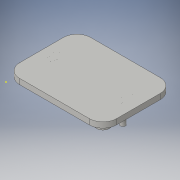
# Autodesk Inventor part: Router Bottom
Saved by Autodesk Inventor 2016 (Build 200138000, 138)
## iProperties
Created: 2016-01-12
Part Number: Router Bottom
Material: Generic
Document SubType Name: Modeling
Designer: Spooner
Density: 1 g/cm^3
Appearance: Default
Author: Spooner
Autodesk Inventor part; units mm, degrees
ref_plane "YZ Plane" through (0, 0, 0) normal (1, 0, 0) x (0, 1, 0)
ref_plane "XZ Plane" through (0, 0, 0) normal (0, 1, 0) x (-1, 0, 0)
ref_plane "XY Plane" through (0, 0, 0) normal (0, 0, 1) x (1, 0, 0)
sketch "Sketch1" plane through (0, 0, 0) normal (0, 1, 0) x (-1, 0, 0)
  line L0 (0, 0) -> (-90.17, 0)
  line L1 (-90.17, 0) -> (-90.17, -66.04)
  line L2 (-90.17, -66.04) -> (0, -66.04)
  line L3 (0, -66.04) -> (0, 0)
  dimension "d0" = 90.17
  dimension "d1" = 66.04
  constraints: 8 end point, 2 parallel, 1 horizontal, 1 perpendicular
  measures "d0" distance of L1.end L2.end
  measures "d1" distance of L0.end L1.end
extrude "Extrusion1" add sketch "Sketch1" along normal blind 5.08
sketch "Sketch2" plane through (0, 0, 0) normal (0, -1, 0) x (1, 0, 0)
  circle A0 centre (8.9218, -8.9217) radius 5.8738
  circle A1 centre (81.2483, -8.9218) radius 5.8738
  circle A2 centre (8.9217, -57.1183) radius 5.8738
  circle A3 centre (81.2483, -57.1183) radius 5.8738
  line L0 (0, 0) -> (90.17, 0) projected
  line L1 (0, -66.04) -> (0, 0) projected
  line L2 (90.17, -66.04) -> (0, -66.04) projected
  line L3 (90.17, 0) -> (90.17, -66.04) projected
  dimension "d4" = 11.7475
  dimension "d5" = 3.048
  dimension "d6" = 3.048
  dimension "d7" = 3.048
  dimension "d8" = 3.048
  constraints: 4 centre point, 3 equal radius, 2 horizontal alignment, 2 vertical alignment
  measures "d4" diameter of A0
  measures "d5" distance edge to line of A1 L0
  measures "d6" distance edge to line of A1 L3
  measures "d7" distance edge to line of A0 L1
  measures "d8" distance edge to line of A3 L2
extrude "Extrusion2" add sketch "Sketch2" along normal blind 2.5908 contours A0 | A1 | A2 | A3
sketch "Sketch3" plane through (0, 0, 0) normal (0, -1, 0) x (1, 0, 0)
  line L0 (78.6638, -30.099) -> (78.6638, -35.941) construction
  line L1 (73.5838, -30.099) -> (73.5838, -35.941)
  line L2 (83.7438, -35.941) -> (83.7438, -30.099)
  arc A0 (83.7438, -30.099) -> (73.5838, -30.099) centre (78.6638, -30.099) ccw
  arc A1 (73.5838, -35.941) -> (83.7438, -35.941) centre (78.6638, -35.941) ccw
  line L3 (11.5062, -30.099) -> (11.5062, -35.941) construction
  line L4 (6.4262, -30.099) -> (6.4262, -35.941)
  line L5 (16.5862, -35.941) -> (16.5862, -30.099)
  arc A2 (16.5862, -30.099) -> (6.4262, -30.099) centre (11.5062, -30.099) ccw
  arc A3 (6.4262, -35.941) -> (16.5862, -35.941) centre (11.5062, -35.941) ccw
  line L6 (90.17, 0) -> (90.17, -66.04) projected
  line L7 (0, -66.04) -> (0, 0) projected
  point P0 (78.6638, -33.02)
  point P1 (11.5062, -33.02)
  point P2 (90.17, -33.02)
  dimension "d11" = 6.4262
  dimension "d12" = 10.16
  dimension "d14" = 6.4262
  dimension "d15" = 16.002
  constraints: 16 end point, 8 point on circle, 8 tangent, 4 centre point, 3 midpoint, 3 parallel, 2 horizontal alignment, 2 vertical, 1 equal radius
  measures "d11" distance from line of L2 point (90.17, -33.02)
  measures "d12" distance from line of L1.end L2
  measures "d14" distance between parallel lines of L4 L7
extrude "Extrusion3" add sketch "Sketch3" along normal blind 4.064
sketch "Sketch4" plane through (0, -4.064, 0) normal (0, -1, 0) x (1, 0, 0)
  point P0 (0, 0)
sketch "Sketch5" plane through (0, -4.064, 0) normal (0, -1, 0) x (1, 0, 0)
  circle A0 centre (78.6638, -35.941) radius 4.1275
  circle A1 centre (11.5062, -35.941) radius 4.1275
  arc A2 (6.4262, -35.941) -> (16.5862, -35.941) centre (11.5062, -35.941) ccw projected
  arc A3 (73.5838, -35.941) -> (83.7438, -35.941) centre (78.6638, -35.941) ccw projected
  line L0 (11.5062, -35.941) -> (11.5062, -30.099) construction
  line L1 (14.4272, -35.941) -> (14.4272, -30.099)
  line L2 (8.5852, -30.099) -> (8.5852, -35.941)
  arc A4 (8.5852, -35.941) -> (14.4272, -35.941) centre (11.5062, -35.941) ccw
  arc A5 (14.4272, -30.099) -> (8.5852, -30.099) centre (11.5062, -30.099) ccw
  line L3 (78.6638, -35.941) -> (78.6638, -30.099) construction
  line L4 (81.5848, -35.941) -> (81.5848, -30.099)
  line L5 (75.7428, -30.099) -> (75.7428, -35.941)
  arc A6 (75.7428, -35.941) -> (81.5848, -35.941) centre (78.6638, -35.941) ccw
  arc A7 (81.5848, -30.099) -> (75.7428, -30.099) centre (78.6638, -30.099) ccw
  arc A8 (16.5862, -30.099) -> (6.4262, -30.099) centre (11.5062, -30.099) ccw projected
  point P0 (0, 0)
  point P1 (11.5062, -33.02)
  point P2 (78.6638, -33.02)
  dimension "d18" = 5.842
  dimension "d19" = 8.255
  constraints: 16 end point, 8 point on circle, 8 tangent, 6 centre point, 4 concentric, 3 parallel, 2 equal radius, 2 midpoint, 2 vertical
  measures "d18" distance between parallel lines of L1 L2
  measures "d19" diameter of A1
extrude "Extrusion4" cut sketch "Sketch5" against normal blind 8.89
fillet "Fillet1" radius 12.7 4 edges at (90.17, 2.54, 0) (90.17, 2.54, -66.04) (0, 2.54, 0) (0, 2.54, -66.04)
sketch "Sketch6" plane through (0, 4.826, 0) normal (0, -1, 0) x (1, 0, 0)
  circle A0 centre (11.5062, -30.099) radius 2.286
  arc A1 (14.4272, -30.099) -> (8.5852, -30.099) centre (11.5062, -30.099) ccw projected
  circle A2 centre (78.6638, -30.099) radius 2.286
  arc A3 (81.5848, -30.099) -> (75.7428, -30.099) centre (78.6638, -30.099) ccw projected
  point P0 (0, 0)
  dimension "d23" = 4.572
  dimension "d24" = 4.572
  constraints: 2 centre point, 2 concentric
  measures "d23" diameter of A0
  measures "d24" diameter of A2
extrude "Extrusion5" add sketch "Sketch6" along normal blind 19.05
equation "\"d6\" = d5"
equation "\"d7\" = d5"
equation "\"d8\" = d5"
equation "\"d14\" = d11"
body "Solid1"
